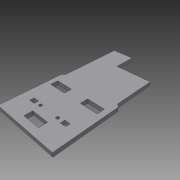
# Autodesk Inventor part: x_carriage_front
Saved by Autodesk Inventor 2014 (Build 180170000, 170)
## iProperties
Created: 2014-02-23
Part Number: x_carriage_front
Material: Generic
Document SubType Name: Modeling
Designer: buben
Density: 1 g/cm^3
Appearance: Default
Author: buben
Autodesk Inventor part; units mm, degrees
ref_plane "YZ Plane" through (0, 0, 0) normal (1, 0, 0) x (0, 1, 0)
ref_plane "XZ Plane" through (0, 0, 0) normal (0, 1, 0) x (-1, 0, 0)
ref_plane "XY Plane" through (0, 0, 0) normal (0, 0, 1) x (1, 0, 0)
sketch "Sketch1" plane through (0, 0, 0) normal (0, 0, 1) x (1, 0, 0)
  line L0 (0, 0) -> (92, 0)
  line L1 (92, 0) -> (92, 87.5)
  line L2 (0, 87.5) -> (0, 0)
  line L3 (0, 87.5) -> (4, 91.5)
  line L4 (92, 87.5) -> (88, 91.5)
  line L5 (4, 91.5) -> (4, 183.5)
  line L6 (88, 91.5) -> (88, 151.5)
  line L7 (34.5, 21) -> (57.5, 21)
  line L8 (58.5, 20) -> (58.5, 11)
  line L9 (57.5, 10) -> (34.5, 10)
  line L10 (33.5, 11) -> (33.5, 20)
  arc A0 (34.5, 21) -> (33.5, 20) centre (34.5, 20) ccw
  arc A1 (33.5, 11) -> (34.5, 10) centre (34.5, 11) ccw
  arc A2 (57.5, 10) -> (58.5, 11) centre (57.5, 11) ccw
  arc A3 (58.5, 20) -> (57.5, 21) centre (57.5, 20) ccw
  line L11 (9, 75) -> (32, 75)
  line L12 (33, 74) -> (33, 65)
  line L13 (32, 64) -> (9, 64)
  line L14 (8, 65) -> (8, 74)
  arc A4 (9, 75) -> (8, 74) centre (9, 74) ccw
  arc A5 (8, 65) -> (9, 64) centre (9, 65) ccw
  arc A6 (32, 64) -> (33, 65) centre (32, 65) ccw
  arc A7 (33, 74) -> (32, 75) centre (32, 74) ccw
  arc A8 (59, 65) -> (60, 64) centre (60, 65) ccw
  arc A9 (60, 75) -> (59, 74) centre (60, 74) ccw
  line L15 (83, 64) -> (60, 64)
  line L16 (84, 74) -> (84, 65)
  arc A10 (83, 64) -> (84, 65) centre (83, 65) ccw
  arc A11 (84, 74) -> (83, 75) centre (83, 74) ccw
  line L17 (60, 75) -> (83, 75)
  line L18 (59, 65) -> (59, 74)
  line L19 (4, 183.5) -> (36, 183.5)
  line L20 (36, 183.5) -> (36, 151.5)
  line L21 (36, 151.5) -> (88, 151.5)
  point P0 (46, 10)
  point P1 (46, 0)
  point P2 (84, 69.5)
  point P3 (58.5, 15.5)
  dimension "d0" = 92
  dimension "d1" = 135
  dimension "d2" = 1
  dimension "d3" = 11
  dimension "d4" = 25
  dimension "d5" = 1
  dimension "d6" = 11
  dimension "d7" = 25
  dimension "d8" = 1
  dimension "d9" = 11
  dimension "d10" = 25
  dimension "d11" = 4
  dimension "d12" = 54
  dimension "d13" = 8
  dimension "d14" = 8
  dimension "d15" = 10
  dimension "d16" = 32
  dimension "d17" = 32
  dimension "d18" = 183.5
  dimension "d19" = 87.5
  constraints: 44 end point, 24 point on circle, 24 tangent, 12 centre point, 11 parallel, 9 equal radius, 6 perpendicular, 4 horizontal, 4 midpoint, 2 horizontal alignment, 1 collinear, 1 vertical alignment
  measures "d0" distance of L0.start L0.end
  measures "d1" angle of L2 L3
  measures "d2" radius of A0
  measures "d3" distance between parallel lines of L9 L7
  measures "d4" distance between parallel lines of L8 L10
  measures "d5" radius of A4
  measures "d6" distance between parallel lines of L13 L11
  measures "d7" distance between parallel lines of L12 L14
  measures "d8" radius of A9
  measures "d9" distance between parallel lines of L15 L17
  measures "d10" distance between parallel lines of L16 L18
  measures "d11" distance between parallel lines of L5 L2
  measures "d12" vertical distance of point (84, 69.5) point (58.5, 15.5)
  measures "d13" distance between parallel lines of L2 L14
  measures "d14" distance between parallel lines of L1 L16
  measures "d15" distance between parallel lines of L0 L9
  measures "d16" distance between parallel lines of L21 L19
  measures "d17" distance of L5.end L19.end
  measures "d18" distance between parallel lines of L0 L19
  measures "d19" distance from line of L2.start L0
extrude "Extrusion1" add sketch "Sketch1" along normal blind 6
sketch "Sketch2" plane through (0, 0, 6) normal (0, 0, 1) x (1, 0, 0)
  line L0 (34.5, 21) -> (57.5, 21) projected
  line L1 (33.5, 11) -> (33.5, 20) projected
  line L2 (34, 23) -> (58, 23) construction
  line L3 (58, 23) -> (58, 8) construction
  line L4 (58, 8) -> (34, 8) construction
  line L5 (34, 8) -> (34, 23) construction
  circle A0 centre (31.75, 32) radius 2.25
  circle A1 centre (60.25, 32) radius 2.25
  line L6 (31.75, 32) -> (60.25, 32) construction
  point P0 (34, 15.5)
  point P1 (33.5, 15.5)
  point P2 (46, 23)
  point P3 (46, 21)
  point P4 (46, 32)
  dimension "d22" = 24
  dimension "d23" = 15
  dimension "d24" = 4.5
  dimension "d25" = 28.5
  dimension "d26" = 9
  constraints: 10 end point, 5 midpoint, 2 centre point, 2 horizontal alignment, 2 parallel, 2 perpendicular, 2 vertical alignment, 1 equal radius, 1 horizontal
  measures "d22" distance between parallel lines of L3 L5
  measures "d23" distance of L2.end L3.end
  measures "d24" diameter of A0
  measures "d25" distance of L6.end L6.start
  measures "d26" distance from line of L2 L6.start
extrude "Extrusion2" cut sketch "Sketch2" against normal blind 6
sketch "Sketch3" plane through (0, 0, 6) normal (0, 0, 1) x (1, 0, 0)
  circle A0 centre (31.75, 32) radius 2.25 projected
  circle A1 centre (60.25, 32) radius 2.25 projected
  line L0 (16.25, 35) -> (24.25, 35)
  line L1 (24.25, 35) -> (24.25, 29)
  line L2 (24.25, 29) -> (16.25, 29)
  line L3 (16.25, 29) -> (16.25, 35)
  line L4 (67.75, 35) -> (75.75, 35)
  line L5 (75.75, 35) -> (75.75, 29)
  line L6 (75.75, 29) -> (67.75, 29)
  line L7 (67.75, 29) -> (67.75, 35)
  point P0 (24.25, 32)
  dimension "d29" = 6
  dimension "d30" = 8
  dimension "d31" = 8
  dimension "d32" = 7.5
  dimension "d33" = 7.5
  constraints: 16 end point, 4 parallel, 2 collinear, 2 horizontal, 2 perpendicular, 1 horizontal alignment, 1 midpoint
  measures "d29" distance of L2.end L0.start
  measures "d30" distance of L0.start L0.end
  measures "d31" distance of L4.start L4.end
  measures "d32" distance from line of A0.centre L1
  measures "d33" distance from line of A1.centre L7
extrude "Extrusion3" cut sketch "Sketch3" against normal blind 6 contours L0 L1 L2 L3 | L4 L5 L6 L7
equation "\"d14\" = d13"
body "Solid1"
